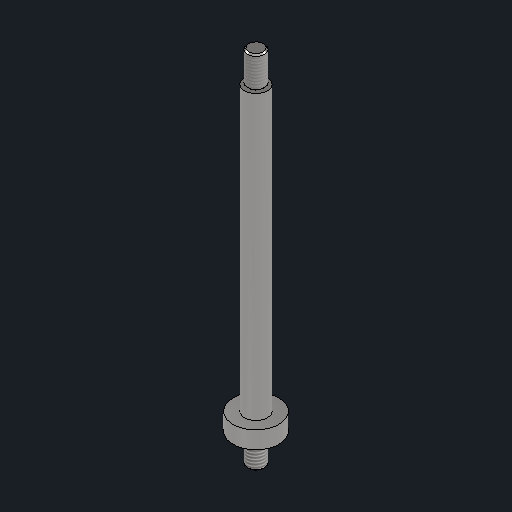
# Autodesk Inventor part: KN-00-02-10
Saved by Autodesk Inventor 2025.2 (Build 292293000, 293)
## iProperties
Created: 2025-04-12
Part Number: KN-00-02-10
Material: X5CrNi18-10
Document SubType Name: Modeling
Designer: Kacper Mik
Density: 8 g/cm^3
Appearance: Semi-Polished
Mass: 12.6648 g
Surface Area: 10.5287 cm^2
Volume: 1.5831 cm^3
Author: Kacper Mik
Autodesk Inventor part; units mm, degrees
ref_plane "YZ Plane" through (0, 0, 0) normal (1, 0, 0) x (0, 1, 0)
ref_plane "XZ Plane" through (0, 0, 0) normal (0, 1, 0) x (-1, 0, 0)
ref_plane "XY Plane" through (0, 0, 0) normal (0, 0, 1) x (1, 0, 0)
sketch "Sketch1" plane through (0, 0, 0) normal (0, 1, 0) x (-1, 0, 0)
  circle A0 centre (0, 0) radius 8
  dimension "d0" = 16
  constraints: 1 centre point, 1 coincident
  measures "d0" diameter of A0
extrude "srodek" add sketch "Sketch1" along normal blind 6
sketch "Sketch2" plane through (0, 0, 0) normal (0, -1, 0) x (1, 0, 0)
  circle A0 centre (0, 0) radius 8 projected
  circle A1 centre (0, 0) radius 3
  dimension "d3" = 6
  constraints: 1 centre point, 1 coincident
  measures "d3" diameter of A1
extrude "dolne" add sketch "Sketch2" along normal blind 10 contours A1
thread "Thread1" size "M6x1" class "6g" standard "ANSI Metric M Profile" full length
chamfer "Chamfer1" distance 0.5 angle 45 1 edges at (-3, -10, 0)
sketch "Sketch3" plane through (0, 0, 0) normal (0, 0, 1) x (1, 0, 0)
  line L0 (3, 0) -> (-3, 0) projected
  line L1 (-3, 0) -> (-2.5, 0)
  line L2 (-2.5, 0) -> (-2.5, -0.5)
  line L3 (-2.5, -0.5) -> (-3, -0.5)
  line L4 (-3, -0.5) -> (-3, 0)
  line L5 (0, -0.6) -> (0, 0.1) projected
  point P0 (0, 0)
  point P1 (-2.5, 0)
  dimension "d11" = 0.5
  dimension "d12" = 0.5
  constraints: 8 end point, 2 parallel, 1 horizontal, 1 perpendicular
  measures "d11" distance of L2.end L3.end
  measures "d12" distance of L1.end L2.end
revolve "Revolution1" cut sketch "Sketch3" angle 360 about axis through (0, -10, 0) along (0, 1, 0)
sketch "Sketch8" plane through (0, 6, 0) normal (0, 1, 0) x (1, 0, 0)
  circle A0 centre (0, 0) radius 4
  dimension "d35" = 8
  constraints: 1 centre point, 1 coincident
  measures "d35" diameter of A0
extrude "gora" add sketch "Sketch8" along normal blind 98.5
sketch "Sketch6" plane through (0, 104.5, 0) normal (0, 1, 0) x (1, 0, 0)
  circle A0 centre (0, 0) radius 4 projected
  circle A1 centre (0, 0) radius 3
  dimension "d19" = 6
  constraints: 1 centre point, 1 coincident
  measures "d19" diameter of A1
extrude "mocowanie K1" add sketch "Sketch6" along normal blind 11 contours A1
thread "Thread3" size "M6x1" class "6g" standard "ISO Metric profile" full length
chamfer "Chamfer3" distance 0.5 angle 45 1 edges at (-3, 115.5, 0)
sketch "Sketch9" plane through (0, 0, 0) normal (0, 0, 1) x (1, 0, 0)
  line L0 (-3, 104.5) -> (3, 104.5) construction
  line L1 (3, 115) -> (-3, 115) construction
  line L2 (3, 104.5) -> (2.5, 104.5)
  line L3 (2.5, 104.5) -> (2.5, 105)
  line L4 (2.5, 105) -> (3, 105)
  line L5 (3, 105) -> (3, 104.5)
  line L6 (0, -35.2) -> (0, 141.2) projected
  point P0 (0, 0)
  dimension "d38" = 0.5
  dimension "d39" = 0.5
  constraints: 8 end point, 2 parallel, 1 horizontal, 1 perpendicular
  measures "d38" distance of L3.end L4.end
  measures "d39" distance of L2.end L3.end
revolve "Revolution3" cut sketch "Sketch9" angle 360 about axis through (0, -10, 0) along (0, 1, 0)
body "Solid1"
